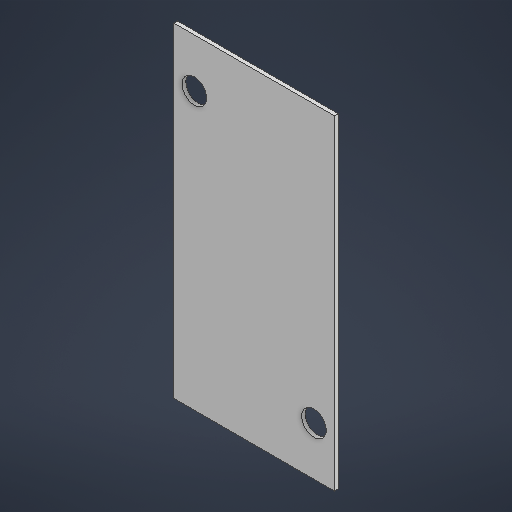
# Autodesk Inventor part: Part1
Saved by Autodesk Inventor 2026.1 (Build 301233020, 233B)
## iProperties
Created: 2026-06-12
Part Number: Part1
Material: Generic
Document SubType Name: Modeling
Designer: Bahaa
Mass: 0.459072 g
Surface Area: 19.1166 cm^2
Volume: 0.459072 cm^3
Density: 1 g/cm^3
Appearance: Default
Author: Bahaa
Autodesk Inventor part; units mm, degrees
ref_plane "YZ Plane" through (0, 0, 0) normal (1, 0, 0) x (0, 1, 0)
ref_plane "XZ Plane" through (0, 0, 0) normal (0, 1, 0) x (-1, 0, 0)
ref_plane "XY Plane" through (0, 0, 0) normal (0, 0, 1) x (1, 0, 0)
sketch "Sketch1" plane through (0, 0, 0) normal (0, 1, 0) x (-1, 0, 0)
  line L0 (10.75, 21.75) -> (-10.75, 21.75)
  line L1 (-10.75, 21.75) -> (-10.75, -21.75)
  line L2 (-10.75, -21.75) -> (10.75, -21.75)
  line L3 (10.75, -21.75) -> (10.75, 21.75)
  line L4 (10.75, 21.75) -> (-10.75, -21.75) construction
  line L5 (-10.75, 21.75) -> (10.75, -21.75) construction
  line L6 (8, -15.25) -> (-8, -15.25) construction
  line L7 (-8, -15.25) -> (-8, 15.25) construction
  line L8 (-8, 15.25) -> (8, 15.25) construction
  line L9 (8, 15.25) -> (8, -15.25) construction
  line L10 (8, -15.25) -> (-8, 15.25) construction
  line L11 (-8, -15.25) -> (8, 15.25) construction
  circle A0 centre (8, 15.25) radius 1.65
  circle A1 centre (-8, -15.25) radius 1.65
  point P0 (0, 0)
  dimension "d0" = 21.5
  dimension "d1" = 43.5
  dimension "d2" = 16
  dimension "d3" = 30.5
  dimension "d4" = 3.3
  dimension "d5" = 3.3
  constraints: 24 end point, 4 midpoint, 4 parallel, 2 centre point, 2 coincident, 2 horizontal, 2 perpendicular
  measures "d0" distance of L2.end L1.end
  measures "d1" distance of L1.end L0.end
  measures "d2" distance of L7.end L8.end
  measures "d3" distance of L6.end L7.end
  measures "d4" diameter of A0
  measures "d5" diameter of A1
extrude "Extrusion1" add sketch "Sketch1" along normal blind 0.5
body "Solid1"
